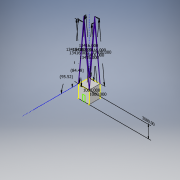
# Autodesk Inventor part: Tower
Saved by Autodesk Inventor 2018 (Build 220112000, 112)
## iProperties
Created: 2019-01-28
Part Number: Tower
Material: Generic
Document SubType Name: Modeling
Designer: This kid
Density: 1 g/cm^3
Appearance: Default
Author: This kid
Autodesk Inventor part; units mm, degrees
ref_plane "YZ Plane" through (0, 0, 0) normal (1, 0, 0) x (0, 1, 0)
ref_plane "XZ Plane" through (0, 0, 0) normal (0, 1, 0) x (-1, 0, 0)
ref_plane "XY Plane" through (0, 0, 0) normal (0, 0, 1) x (1, 0, 0)
sketch "Sketch1" plane through (0, 0, 0) normal (0, 1, 0) x (-1, 0, 0)
  point P0 (0, 0)
sketch "Sketch2" plane through (0, 0, 0) normal (0, 1, 0) x (-1, 0, 0)
  line L0 (0, 0) -> (65532, 0)
  line L1 (65532, 0) -> (65532, -65532)
  line L2 (65532, -65532) -> (0, -65532)
  line L3 (0, -65532) -> (0, 0)
  dimension "d0" = 65532
  dimension "d1" = 65532
  constraints: 8 end point, 2 parallel, 1 horizontal, 1 perpendicular
  measures "d0" distance of L1.end L2.end
  measures "d1" distance of L0.end L1.end
extrude "Extrusion1" add sketch "Sketch2" along normal blind 76200
sketch "Sketch4" plane through (-65532, 0, -65532) normal (-1, 0, 0) x (0, 0, 1)
  line L0 (15240, 0) -> (50292, 0)
  line L1 (50292, 0) -> (50292, 36231.95)
  line L2 (50292, 36231.95) -> (15240, 36231.95)
  line L3 (15240, 36231.95) -> (15240, 0)
  line L4 (0, 0) -> (0, 76200) projected
  line L5 (65532, 0) -> (65532, 76200) projected
  dimension "d12" = 15240
  dimension "d13" = 15240
  constraints: 8 end point, 2 parallel, 1 horizontal, 1 perpendicular
  measures "d12" distance between parallel lines of L3 L4
  measures "d13" distance between parallel lines of L1 L5
sketch "Sketch5" plane through (0, 0, -65532) normal (0, 0, -1) x (-1, 0, 0)
  line L0 (25400, 0) -> (40132, 0)
  line L1 (40132, 0) -> (40132, 36231.95)
  line L2 (40132, 36231.95) -> (25400, 36231.95)
  line L3 (25400, 36231.95) -> (25400, 0)
  line L4 (0, 0) -> (0, 76200) projected
  line L5 (65532, 0) -> (65532, 76200) projected
  dimension "d16" = 25400
  dimension "d17" = 25400
  constraints: 8 end point, 2 parallel, 1 horizontal, 1 perpendicular
  measures "d16" distance between parallel lines of L4 L3
  measures "d17" distance between parallel lines of L1 L5
sketch "Sketch6" plane through (-65532, 0, 0) normal (0, 0, 1) x (1, 0, 0)
  line L0 (25400, 0) -> (40132, 0)
  line L1 (40132, 0) -> (40132, 36231.95)
  line L2 (40132, 36231.95) -> (25400, 36231.95)
  line L3 (25400, 36231.95) -> (25400, 0)
  constraints: 8 end point, 2 parallel, 1 horizontal, 1 perpendicular
extrude "Extrusion2" cut sketch "Sketch4" against normal blind 2540
ref_plane "Work Plane1" through (0, 76200, 0) normal (0, 0, 1) x (1, 0, 0)
sketch "Sketch7" plane through (0, 76200, 0) normal (0, 0, 1) x (1, 0, 0)
  line L0 (-65532, 0) -> (0, 0) projected
  line L1 (0, 0) -> (-32766, 339187.4535)
  line L2 (-65532, -76200) -> (-65532, 0) projected
  line L3 (-65532, 0) -> (-32766, 339187.4535)
  point P0 (0, -76200)
  dimension "d31" = 340766.4
  dimension "d32" = 340766.4
  constraints: 4 end point
  measures "d31" distance of L0.end L1.end
  measures "d32" distance of L1.end L0.start
ref_plane "Work Plane2" through (-65532, 0, -65532) normal (0, 0, -1) x (0, 1, 0)
ref_plane "Work Plane3" through (0, 76200, -32766) normal (1, 0, 0) x (0, 0, -1)
sketch "Sketch8" plane through (0, 76200, -32766) normal (1, 0, 0) x (0, 0, -1)
  line L0 (-32766, -76200) -> (-32766, 0) projected
  line L1 (-32766, 0) -> (0, 339187.4535)
  line L2 (32766, -76200) -> (32766, 0) projected
  line L3 (32766, 0) -> (0, 339187.4535)
  dimension "d34" = 340766.4
  dimension "d35" = 340766.4
  constraints: 4 end point
  measures "d34" distance of L1.end L0.end
  measures "d35" distance of L2.end L1.end
sketch "Sketch9" plane through (-65532, 0, -65532) normal (0, 0, -1) x (0, 1, 0)
  line L0 (76200, 0) -> (76200, 65532) projected
  line L1 (76200, 65532) -> (415387.4535, 32766)
  line L2 (76200, 0) -> (415387.4535, 32766)
  line L3 (76200, 0) -> (416966.4, 0) construction
  point P0 (0, 65532)
  dimension "d36" = 340766.4
  dimension "d37" = 340766.4
  constraints: 6 end point, 1 horizontal
  measures "d36" distance of L1.end L0.end
  measures "d37" distance of L0.start L1.end
ref_plane "Work Plane4" through (-65532, 0, -7620) normal (-1, 0, 0) x (0, 0, 1)
sketch "Sketch10" plane through (-65532, 0, -7620) normal (-1, 0, 0) x (0, 0, 1)
  line L0 (-57912, 76200) -> (7620, 76200) projected
  line L1 (-57912, 76200) -> (-25146, 415387.4535)
  line L2 (-57912, 76200) -> (282854.4, 76200) construction
  line L3 (7620, 76200) -> (-25146, 415387.4535)
  line L4 (7620, 76200) -> (348386.4, 76200) construction
  point P0 (7620, 0)
  dimension "d39" = 340766.4
  dimension "d40" = 84.482
  dimension "d41" = 340766.4
  dimension "d42" = 95.518
  constraints: 8 end point, 2 horizontal
  measures "d39" distance of L1.end L0.start
  measures "d40" angle of L2 L1
  measures "d41" distance of L0.end L1.end
  measures "d42" angle of L4 L3
body "Solid1"
